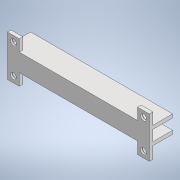
# Autodesk Inventor part: RackSlider
Saved by Autodesk Inventor 2022 (Build 260153000, 153)
## iProperties
Created: 2022-06-04
Part Number: RackSlider
Material: Generic
Document SubType Name: Modeling
Designer: frede
Density: 1 g/cm^3
Appearance: Default
Author: frede
Autodesk Inventor part; units mm, degrees
ref_plane "YZ Plane" through (0, 0, 0) normal (1, 0, 0) x (0, 1, 0)
ref_plane "XZ Plane" through (0, 0, 0) normal (0, 1, 0) x (-1, 0, 0)
ref_plane "XY Plane" through (0, 0, 0) normal (0, 0, 1) x (1, 0, 0)
sketch "Sketch1" plane through (0, 0, 0) normal (1, 0, 0) x (0, 1, 0)
  line L0 (-3.8911, -13.4939) -> (4.1089, -13.4939) construction
  line L1 (4.1089, -13.4939) -> (4.1089, 2.1061) construction
  line L2 (4.1089, 2.1061) -> (-3.8911, 2.1061) construction
  line L3 (-3.8911, 2.1061) -> (-3.8911, -13.4939) construction
  line L4 (10.4519, -45.082) -> (10.4519, -29.482) construction
  line L5 (10.4519, -45.082) -> (2.4519, -45.082) construction
  line L6 (2.4519, -29.482) -> (2.4519, -45.082) construction
  line L7 (10.4519, -29.482) -> (2.4519, -29.482) construction
  line L8 (4.6089, -13.9939) -> (4.6089, 2.6061)
  line L9 (4.6089, 2.6061) -> (-4.3911, 2.6061)
  line L10 (-4.3911, 2.6061) -> (-4.3911, -13.9939)
  line L11 (7.6089, -13.9939) -> (7.6089, 5.6061)
  line L12 (7.6089, 5.6061) -> (-7.3911, 5.6061)
  line L13 (-7.3911, 5.6061) -> (-7.3911, -13.9939)
  line L14 (-7.3911, -13.9939) -> (-4.3911, -13.9939)
  line L15 (4.6089, -13.9939) -> (7.6089, -13.9939)
  point P0 (0, 0)
  dimension "d1" = 0.5
  dimension "d2" = 3
  constraints: 24 end point, 6 parallel, 3 horizontal, 2 horizontal alignment, 1 perpendicular, 4 other
  measures "d1" distance between parallel lines of L3 L10
  measures "d2" distance between parallel lines of L10 L13
extrude "Extrusion1" add sketch "Sketch1" along normal blind 120
sketch "Sketch2" plane through (0, -7.3911, -13.9939) normal (0, -1, 0) x (1, 0, 0)
  line L0 (0, 19.6) -> (0, 0) projected
  line L1 (0, 19.6) -> (10, 19.6)
  line L2 (10, 19.6) -> (10, 16.6)
  line L3 (10, 16.6) -> (0, 16.6)
  line L4 (0, 16.6) -> (0, 19.6)
  line L5 (0, 19.6) -> (120, 19.6) projected
  line L6 (120, 19.6) -> (110, 19.6)
  line L7 (110, 19.6) -> (110, 16.6)
  line L8 (110, 16.6) -> (120, 16.6)
  line L9 (120, 16.6) -> (120, 19.6)
  point P0 (0, 13.9939)
  point P1 (110, 19.6)
  dimension "d5" = 10
  dimension "d6" = 3
  dimension "d7" = 10
  dimension "d8" = 3
  constraints: 16 end point, 4 parallel, 2 horizontal, 2 perpendicular
  measures "d5" distance of L2.end L3.end
  measures "d6" distance of L1.end L2.end
  measures "d7" distance of L8.end L7.end
  measures "d8" distance of L7.end L6.end
extrude "Extrusion2" add sketch "Sketch2" along normal blind 10
sketch "Sketch4" plane through (10, -7.3911, 2.6061) normal (0, 0, -1) x (-1, 0, 0)
  circle A0 centre (5, -5) radius 2.5
  line L0 (0, 0) -> (0, -10) projected
  line L1 (10, -10) -> (0, -10) projected
  circle A1 centre (-105, -5) radius 2.5
  line L2 (-110, 0) -> (-110, -10) projected
  line L3 (-100, -10) -> (-110, -10) projected
  point P0 (10, 7.3911)
  point P1 (0, -5)
  point P2 (5, -10)
  point P3 (-110, -5)
  point P4 (-105, -10)
  dimension "d11" = 5
  dimension "d12" = 5
  constraints: 4 midpoint, 2 centre point, 2 horizontal alignment, 2 vertical alignment
  measures "d11" diameter of A0
  measures "d12" diameter of A1
extrude "Extrusion3" cut sketch "Sketch4" against normal through all
chamfer "Chamfer1" distance 1.5 angle 45 2 edges at (7.5, -12.3911, 2.6061) (117.5, -12.3911, 2.6061)
mirror "Mirror1" about plane through (0, 0, 0) normal (0, 1, 0) of "Extrusion2", "Extrusion3", "Chamfer1"
body "Solid1"
